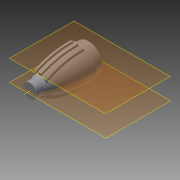
# Autodesk Inventor part: Mufflertip
Saved by Autodesk Inventor 2015 (Build 190159000, 159)
## iProperties
Created: 2016-02-28
Part Number: Mufflertip
Material: Generic
Document SubType Name: Modeling
Designer: Owner
Density: 1 g/cm^3
Appearance: Default
Mass: 6.07664 g
Surface Area: 88.6231 cm^2
Volume: 6.07664 cm^3
Author: Owner
Autodesk Inventor part; units mm, degrees
ref_plane "YZ Plane" through (0, 0, 0) normal (1, 0, 0) x (0, 1, 0)
ref_plane "XY Plane" through (0, 0, 0) normal (0, 0, 1) x (1, 0, 0)
sketch "Sketch1" plane through (0, 0, 0) normal (0, 1, 0) x (-1, 0, 0)
  line L0 (44.1059, -32.7618) -> (43.305, -25.1418)
  arc A0 (50.2079, 14.2711) -> (42.035, -20.0618) centre (118.235, -20.0618) ccw
  line L1 (50.2079, 14.2711) -> (50.2079, 20.6211)
  line L2 (50.2079, 20.6211) -> (56.5579, 20.6211)
  line L3 (56.5579, 20.6211) -> (56.5579, -25.1418)
  line L4 (56.5579, -25.1418) -> (56.5579, -32.7618)
  line L5 (56.5579, -32.7618) -> (44.1059, -32.7618)
  line L6 (42.035, -20.0618) -> (42.035, -25.1418)
  line L7 (42.035, -25.1418) -> (43.305, -25.1418)
  point P0 (0, 0)
  dimension "d0" = 76.2
  dimension "d1" = 6.35
  dimension "d2" = 6.35
  dimension "d3" = 5.08
  dimension "d4" = 1.27
  dimension "d5" = 13.2528
  dimension "d6" = 6
  dimension "d7" = 7.62
  constraints: 16 end point, 4 perpendicular, 2 point on circle, 1 centre point, 1 collinear, 1 parallel, 1 tangent
  measures "d0" radius of A0
  measures "d1" distance of L1.start L1.end
  measures "d2" distance of L1.end L2.end
  measures "d3" distance of L6.start L6.end
  measures "d4" distance of L6.end L0.end
  measures "d5" distance from line of L0.end L3
  measures "d6" angle of L6 L0
  measures "d7" distance between parallel lines of L7 L5
revolve "Revolution1" add sketch "Sketch1" angle 360 about axis through (-56.5579, 0, 20.6211) along (0, 0, -1)
shell "Shell1" thickness 1.27 removed faces 1 at (-53.3304, 3.7457, -32.7618)
ref_plane "Work Plane1" through (0, 19.05, 0) normal (0, 1, 0) x (-1, 0, 0)
sketch "Sketch2" plane through (0, 19.05, 0) normal (0, 1, 0) x (-1, 0, 0)
  line L0 (71.0807, -20.0618) -> (42.035, -20.0618) projected
  line L1 (62.9079, 14.2711) -> (50.2079, 14.2711) projected
  line L2 (62.9079, 14.2711) -> (50.2079, 14.2711) projected
  line L3 (62.9079, 20.6211) -> (50.2079, 20.6211) projected
  line L4 (69.0098, -32.7618) -> (44.1059, -32.7618) projected
  line L5 (69.8107, -25.1418) -> (43.305, -25.1418) projected
  arc A0 (71.0807, -20.0618) -> (62.9079, 14.2711) centre (-5.1193, -20.0618) ccw projected
  arc A1 (50.2079, 14.2711) -> (42.035, -20.0618) centre (118.235, -20.0618) ccw projected
  line L6 (56.5579, 20.6211) -> (56.5579, -32.7618) construction
  line L7 (56.5579, 11.7311) -> (57.8279, 11.7311) construction
  line L8 (57.8279, 11.7311) -> (55.2879, 11.7311)
  line L9 (55.2879, 11.7311) -> (55.2879, -22.6097)
  line L10 (55.2879, -22.6097) -> (57.8279, -22.6097)
  line L11 (57.8279, -22.6097) -> (57.8279, 11.7311)
  line L12 (57.8279, 11.7311) -> (60.3679, 11.7311) construction
  line L13 (60.3679, 11.7311) -> (62.9079, 11.7311)
  line L14 (62.9079, 11.7311) -> (62.9079, -22.6097)
  line L15 (62.9079, -22.6097) -> (60.3679, -22.6097)
  line L16 (60.3679, -22.6097) -> (60.3679, 11.7311)
  line L17 (55.2879, 11.7311) -> (52.7479, 11.7311) construction
  line L18 (52.7479, 11.7311) -> (50.2079, 11.7311)
  line L19 (50.2079, 11.7311) -> (50.2079, -22.6097)
  line L20 (50.2079, -22.6097) -> (52.7479, -22.6097)
  line L21 (52.7479, -22.6097) -> (52.7479, 11.7311)
  point P0 (0, 0)
  dimension "d11" = 1.27
  dimension "d12" = 2.54
  dimension "d13" = 2.54
  dimension "d14" = 34.3408
  dimension "d15" = 2.54
  dimension "d16" = 2.54
  constraints: 32 end point, 6 parallel, 5 horizontal, 4 perpendicular, 2 midpoint, 1 point on line
  measures "d11" distance of L7.start L7.end
  measures "d12" distance between parallel lines of L1 L7
  measures "d13" distance of L10.end L9.end
  measures "d14" distance of L9.end L8.end
  measures "d15" distance of L7.end L12.end
  measures "d16" distance of L8.end L17.end
emboss "Emboss1" sketch "Sketch2" operation add depth 1.905 direction (0, -1, 0) contours L14 L15 L16 L0 | L0 L16 L13 L14 | L11 L10 L9 L0 | L0 L9 L8 L11 | L19 L18 L21 L0 | L0 L21 L20 L19
fillet "Fillet1" radius 0.635 12 edges at (-50.2079, 5.7064, 11.7311) (-52.7479, 7.7135, 11.7311) (-55.2879, 8.5234, 11.7311) (-62.9079, 5.7064, 11.7311) (-60.3679, 7.7135, 11.7311) (-56.5579, 9.6643, 11.7311) (-50.2079, 14.106, -22.6097) (-52.7479, 14.997, -22.6097) (-55.2879, 15.4229, -22.6097) (-57.8279, 15.4229, -22.6097) (-60.3679, 14.997, -22.6097) (-62.9079, 14.106, -22.6097)
mirror "Mirror1" about plane through (0, 0, 0) normal (0, 1, 0) of "Emboss1"
equation "\"d2\" = d1"
body "Solid1"
